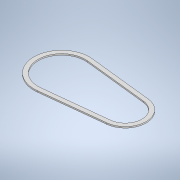
# Autodesk Inventor part: Dichtungsgummi
Saved by Autodesk Inventor 2021 (Build 250183000, 183)
## iProperties
Created: 2021-01-19
Part Number: Dichtungsgummi
Material: Generisch
Document SubType Name: Modeling
Designer: Jaro Machnow
Density: 1 g/cm^3
Appearance: Vorgabe
Author: Jaro Machnow
Autodesk Inventor part; units mm, degrees
ref_plane "YZ Plane" through (0, 0, 0) normal (1, 0, 0) x (0, 1, 0)
ref_plane "XZ Plane" through (0, 0, 0) normal (0, 1, 0) x (-1, 0, 0)
ref_plane "XY Plane" through (0, 0, 0) normal (0, 0, 1) x (1, 0, 0)
sketch "Skizze1" plane through (0, 0, 0) normal (0, 1, 0) x (-1, 0, 0)
  arc A0 (-2.1739, -19.8815) -> (-2.1739, 19.8815) centre (0, 0) ccw
  arc A1 (-47.6304, 14.9111) -> (-47.6304, -14.9111) centre (-46, 0) ccw
  line L0 (-2.1739, 19.8815) -> (-47.6304, 14.9111)
  line L1 (-2.1739, -19.8815) -> (-47.6304, -14.9111)
  line L2 (45.0235, 0) -> (-115.148, 0) construction
  arc A2 (-1.8478, -16.8993) -> (-1.8478, 16.8993) centre (0, 0) ccw
  arc A3 (-47.3043, 11.9289) -> (-47.3043, -11.9289) centre (-46, 0) ccw
  line L3 (-1.8478, 16.8993) -> (-47.3043, 11.9289)
  line L4 (-1.8478, -16.8993) -> (-47.3043, -11.9289)
  dimension "d0" = 40
  dimension "d1" = 30
  dimension "d2" = 46
  dimension "d3" = 3
  dimension "d4" = 3
  constraints: 10 end point, 8 point on circle, 8 tangent, 4 centre point, 4 coincident, 2 horizontal, 1 point on line
  measures "d0" diameter of A0
  measures "d1" diameter of A1
  measures "d2" distance of A1.centre point (0, 0)
  measures "d3" radial gap between concentric circles of A0 A2
  measures "d4" radial gap between concentric circles of A1 A3
extrude "Extrusion1" add sketch "Skizze1" along normal blind 1
